Autodesk Inventor part; units mm, degrees
(part 2 of 2)
  line L957 (3.5682, -5.3852) -> (3.5463, -5.3913)
  line L958 (3.5463, -5.3913) -> (3.5215, -5.4036)
  line L959 (3.5215, -5.4036) -> (3.2974, -5.5433)
  line L960 (3.2974, -5.5433) -> (3.2248, -5.5858)
  line L961 (3.2248, -5.5858) -> (3.1517, -5.6274)
  line L962 (3.1517, -5.6274) -> (2.9187, -5.7518)
  line L963 (2.9187, -5.7518) -> (2.8957, -5.7671)
  line L964 (2.8957, -5.7671) -> (2.8794, -5.783)
  line L965 (2.8794, -5.783) -> (2.8651, -5.8021)
  line L966 (2.8651, -5.8021) -> (2.8529, -5.8243)
  line L967 (2.8529, -5.8243) -> (2.843, -5.8495)
  line L968 (2.843, -5.8495) -> (2.8303, -5.9087)
  line L969 (2.8303, -5.9087) -> (2.8281, -5.9788)
  line L970 (2.8281, -5.9788) -> (2.8371, -6.0592)
  line L971 (2.8371, -6.0592) -> (2.8582, -6.1489)
  line L972 (2.8582, -6.1489) -> (2.8922, -6.2471)
  line L973 (2.8922, -6.2471) -> (2.9398, -6.3529)
  line L974 (2.9398, -6.3529) -> (2.9659, -6.4039)
  line L975 (2.9659, -6.4039) -> (2.9967, -6.501)
  line L976 (2.9967, -6.501) -> (3.0239, -6.628)
  line L977 (3.0239, -6.628) -> (3.0364, -6.7098)
  line L978 (3.0364, -6.7098) -> (3.0468, -6.8051)
  line L979 (3.0468, -6.8051) -> (3.0541, -6.9129)
  line L980 (3.0541, -6.9129) -> (3.0571, -7.033)
  line L981 (3.0571, -7.033) -> (3.0548, -7.1683)
  line L982 (3.0548, -7.1683) -> (3.0464, -7.3121)
  line L983 (3.0464, -7.3121) -> (3.0306, -7.4689)
  line L984 (3.0306, -7.4689) -> (3.0065, -7.6369)
  line L985 (3.0065, -7.6369) -> (2.9731, -7.8164)
  line L986 (2.9731, -7.8164) -> (2.9366, -7.9766)
  arc A18 (2.3128, -8.1793) -> (2.9366, -7.9766) centre (0, 0) ccw
  line L987 (2.3128, -8.1793) -> (2.1908, -8.0711)
  line L988 (2.1908, -8.0711) -> (2.0582, -7.9456)
  line L989 (2.0582, -7.9456) -> (1.94, -7.8238)
  line L990 (1.94, -7.8238) -> (1.835, -7.7062)
  line L991 (1.835, -7.7062) -> (1.7437, -7.5949)
  line L992 (1.7437, -7.5949) -> (1.6623, -7.4867)
  line L993 (1.6623, -7.4867) -> (1.5942, -7.3878)
  line L994 (1.5942, -7.3878) -> (1.5367, -7.2963)
  line L995 (1.5367, -7.2963) -> (1.4891, -7.2131)
  line L996 (1.4891, -7.2131) -> (1.4511, -7.1396)
  line L997 (1.4511, -7.1396) -> (1.3985, -7.0209)
  line L998 (1.3985, -7.0209) -> (1.3663, -6.9242)
  line L999 (1.3663, -6.9242) -> (1.3573, -6.8676)
  line L1000 (1.3573, -6.8676) -> (1.3337, -6.754)
  line L1001 (1.3337, -6.754) -> (1.3034, -6.6546)
  line L1002 (1.3034, -6.6546) -> (1.2678, -6.5696)
  line L1003 (1.2678, -6.5696) -> (1.2278, -6.4993)
  line L1004 (1.2278, -6.4993) -> (1.1847, -6.4439)
  line L1005 (1.1847, -6.4439) -> (1.1397, -6.4035)
  line L1006 (1.1397, -6.4035) -> (1.1169, -6.389)
  line L1007 (1.1169, -6.389) -> (1.094, -6.3782)
  line L1008 (1.094, -6.3782) -> (1.0712, -6.3711)
  line L1009 (1.0712, -6.3711) -> (1.0486, -6.3678)
  line L1010 (1.0486, -6.3678) -> (1.021, -6.369)
  line L1011 (1.021, -6.369) -> (0.7594, -6.4054)
  line L1012 (0.7594, -6.4054) -> (0.6758, -6.4147)
  line L1013 (0.6758, -6.4147) -> (0.5922, -6.423)
  line L1014 (0.5922, -6.423) -> (0.3287, -6.4418)
  line L1015 (0.3287, -6.4418) -> (0.3014, -6.4464)
  line L1016 (0.3014, -6.4464) -> (0.2801, -6.4543)
  line L1017 (0.2801, -6.4543) -> (0.2592, -6.4659)
  line L1018 (0.2592, -6.4659) -> (0.2391, -6.4813)
  line L1019 (0.2391, -6.4813) -> (0.2197, -6.5002)
  line L1020 (0.2197, -6.5002) -> (0.1841, -6.5491)
  line L1021 (0.1841, -6.5491) -> (0.1535, -6.6123)
  line L1022 (0.1535, -6.6123) -> (0.1291, -6.6893)
  line L1023 (0.1291, -6.6893) -> (0.1119, -6.7799)
  line L1024 (0.1119, -6.7799) -> (0.103, -6.8834)
  line L1025 (0.103, -6.8834) -> (0.1034, -6.9994)
  line L1026 (0.1034, -6.9994) -> (0.1065, -7.0567)
  line L1027 (0.1065, -7.0567) -> (0.0951, -7.1579)
  line L1028 (0.0951, -7.1579) -> (0.0683, -7.285)
  line L1029 (0.0683, -7.285) -> (0.0464, -7.3648)
  line L1030 (0.0464, -7.3648) -> (0.0172, -7.4561)
  line L1031 (0.0172, -7.4561) -> (-0.02, -7.5575)
  line L1032 (-0.02, -7.5575) -> (-0.0661, -7.6685)
  line L1033 (-0.0661, -7.6685) -> (-0.1232, -7.7912)
  line L1034 (-0.1232, -7.7912) -> (-0.1894, -7.919)
  line L1035 (-0.1894, -7.919) -> (-0.2676, -8.0559)
  line L1036 (-0.2676, -8.0559) -> (-0.3579, -8.1996)
  line L1037 (-0.3579, -8.1996) -> (-0.4615, -8.35)
  line L1038 (-0.4615, -8.35) -> (-0.5599, -8.4815)
  arc A19 (-1.2139, -8.4129) -> (-0.5599, -8.4815) centre (0, 0) ccw
  line L1039 (-1.2139, -8.4129) -> (-1.283, -8.2636)
  line L1040 (-1.283, -8.2636) -> (-1.353, -8.0949)
  line L1041 (-1.353, -8.0949) -> (-1.4115, -7.9356)
  line L1042 (-1.4115, -7.9356) -> (-1.4595, -7.7855)
  line L1043 (-1.4595, -7.7855) -> (-1.4977, -7.6466)
  line L1044 (-1.4977, -7.6466) -> (-1.528, -7.5147)
  line L1045 (-1.528, -7.5147) -> (-1.55, -7.3966)
  line L1046 (-1.55, -7.3966) -> (-1.5653, -7.2897)
  line L1047 (-1.5653, -7.2897) -> (-1.5749, -7.1943)
  line L1048 (-1.5749, -7.1943) -> (-1.5798, -7.1116)
  line L1049 (-1.5798, -7.1116) -> (-1.5796, -6.9818)
  line L1050 (-1.5796, -6.9818) -> (-1.5697, -6.8804)
  line L1051 (-1.5697, -6.8804) -> (-1.5548, -6.8251)
  line L1052 (-1.5548, -6.8251) -> (-1.5302, -6.7117)
  line L1053 (-1.5302, -6.7117) -> (-1.5174, -6.6086)
  line L1054 (-1.5174, -6.6086) -> (-1.5154, -6.5164)
  line L1055 (-1.5154, -6.5164) -> (-1.5234, -6.4359)
  line L1056 (-1.5234, -6.4359) -> (-1.5402, -6.3678)
  line L1057 (-1.5402, -6.3678) -> (-1.5649, -6.3126)
  line L1058 (-1.5649, -6.3126) -> (-1.5798, -6.29)
  line L1059 (-1.5798, -6.29) -> (-1.5964, -6.2708)
  line L1060 (-1.5964, -6.2708) -> (-1.6143, -6.2551)
  line L1061 (-1.6143, -6.2551) -> (-1.6336, -6.2429)
  line L1062 (-1.6336, -6.2429) -> (-1.6593, -6.2328)
  line L1063 (-1.6593, -6.2328) -> (-1.9131, -6.1596)
  line L1064 (-1.9131, -6.1596) -> (-1.9932, -6.1342)
  line L1065 (-1.9932, -6.1342) -> (-2.073, -6.1077)
  line L1066 (-2.073, -6.1077) -> (-2.3214, -6.0177)
  line L1067 (-2.3214, -6.0177) -> (-2.3482, -6.0109)
  line L1068 (-2.3482, -6.0109) -> (-2.3709, -6.0094)
  line L1069 (-2.3709, -6.0094) -> (-2.3947, -6.0116)
  line L1070 (-2.3947, -6.0116) -> (-2.4193, -6.0174)
  line L1071 (-2.4193, -6.0174) -> (-2.4447, -6.0269)
  line L1072 (-2.4447, -6.0269) -> (-2.4971, -6.057)
  line L1073 (-2.4971, -6.057) -> (-2.5507, -6.1023)
  line L1074 (-2.5507, -6.1023) -> (-2.6044, -6.1627)
  line L1075 (-2.6044, -6.1627) -> (-2.657, -6.2385)
  line L1076 (-2.657, -6.2385) -> (-2.7072, -6.3295)
  line L1077 (-2.7072, -6.3295) -> (-2.7539, -6.4356)
  line L1078 (-2.7539, -6.4356) -> (-2.7745, -6.4891)
  line L1079 (-2.7745, -6.4891) -> (-2.826, -6.577)
  line L1080 (-2.826, -6.577) -> (-2.9021, -6.6822)
  line L1081 (-2.9021, -6.6822) -> (-2.9546, -6.7462)
  line L1082 (-2.9546, -6.7462) -> (-3.0185, -6.8178)
  line L1083 (-3.0185, -6.8178) -> (-3.0937, -6.8953)
  line L1084 (-3.0937, -6.8953) -> (-3.1809, -6.9779)
  line L1085 (-3.1809, -6.9779) -> (-3.283, -7.0668)
  line L1086 (-3.283, -7.0668) -> (-3.3955, -7.1566)
  line L1087 (-3.3955, -7.1566) -> (-3.5226, -7.2499)
  line L1088 (-3.5226, -7.2499) -> (-3.6636, -7.3444)
  line L1089 (-3.6636, -7.3444) -> (-3.8194, -7.4396)
  line L1090 (-3.8194, -7.4396) -> (-3.9628, -7.5197)
  arc A20 (-4.5309, -7.1917) -> (-3.9628, -7.5197) centre (0, 0) ccw
  line L1091 (-4.5309, -7.1917) -> (-4.5332, -7.0275)
  line L1092 (-4.5332, -7.0275) -> (-4.5286, -6.8449)
  line L1093 (-4.5286, -6.8449) -> (-4.5172, -6.6756)
  line L1094 (-4.5172, -6.6756) -> (-4.5001, -6.5189)
  line L1095 (-4.5001, -6.5189) -> (-4.4785, -6.3766)
  line L1096 (-4.4785, -6.3766) -> (-4.4526, -6.2437)
  line L1097 (-4.4526, -6.2437) -> (-4.4246, -6.1269)
  line L1098 (-4.4246, -6.1269) -> (-4.3951, -6.023)
  line L1099 (-4.3951, -6.023) -> (-4.3651, -5.9319)
  line L1100 (-4.3651, -5.9319) -> (-4.3359, -5.8544)
  line L1101 (-4.3359, -5.8544) -> (-4.2829, -5.7359)
  line L1102 (-4.2829, -5.7359) -> (-4.2326, -5.6473)
  line L1103 (-4.2326, -5.6473) -> (-4.1965, -5.6028)
  line L1104 (-4.1965, -5.6028) -> (-4.1279, -5.5092)
  line L1105 (-4.1279, -5.5092) -> (-4.0742, -5.4202)
  line L1106 (-4.0742, -5.4202) -> (-4.035, -5.3369)
  line L1107 (-4.035, -5.3369) -> (-4.0094, -5.2601)
  line L1108 (-4.0094, -5.2601) -> (-3.9971, -5.1911)
  line L1109 (-3.9971, -5.1911) -> (-3.9966, -5.1312)
  line L1110 (-3.9966, -5.1312) -> (-4.001, -5.1045)
  line L1111 (-4.001, -5.1045) -> (-4.0083, -5.0803)
  line L1112 (-4.0083, -5.0803) -> (-4.0184, -5.0586)
  line L1113 (-4.0184, -5.0586) -> (-4.031, -5.0396)
  line L1114 (-4.031, -5.0396) -> (-4.0503, -5.0199)
  line L1115 (-4.0503, -5.0199) -> (-4.2524, -4.8498)
  line L1116 (-4.2524, -4.8498) -> (-4.3153, -4.794)
  line L1117 (-4.3153, -4.794) -> (-4.3774, -4.7373)
  line L1118 (-4.3774, -4.7373) -> (-4.5677, -4.5541)
  line L1119 (-4.5677, -4.5541) -> (-4.5893, -4.5369)
  line L1120 (-4.5893, -4.5369) -> (-4.6095, -4.5264)
  line L1121 (-4.6095, -4.5264) -> (-4.6321, -4.5187)
  line L1122 (-4.6321, -4.5187) -> (-4.657, -4.5139)
  line L1123 (-4.657, -4.5139) -> (-4.684, -4.5123)
  line L1124 (-4.684, -4.5123) -> (-4.7442, -4.5185)
  line L1125 (-4.7442, -4.5185) -> (-4.8116, -4.538)
  line L1126 (-4.8116, -4.538) -> (-4.8852, -4.5714)
  line L1127 (-4.8852, -4.5714) -> (-4.964, -4.6192)
  line L1128 (-4.964, -4.6192) -> (-5.0469, -4.6819)
  line L1129 (-5.0469, -4.6819) -> (-5.1328, -4.7599)
  line L1130 (-5.1328, -4.7599) -> (-5.1733, -4.8004)
  line L1131 (-5.1733, -4.8004) -> (-5.2562, -4.8597)
  line L1132 (-5.2562, -4.8597) -> (-5.3685, -4.9249)
  line L1133 (-5.3685, -4.9249) -> (-5.4425, -4.962)
  line L1134 (-5.4425, -4.962) -> (-5.5299, -5.0014)
  line L1135 (-5.5299, -5.0014) -> (-5.6301, -5.0416)
  line L1136 (-5.6301, -5.0416) -> (-5.7434, -5.0816)
  line L1137 (-5.7434, -5.0816) -> (-5.8728, -5.1213)
  line L1138 (-5.8728, -5.1213) -> (-6.0121, -5.1577)
  line L1139 (-6.0121, -5.1577) -> (-6.1662, -5.1911)
  line L1140 (-6.1662, -5.1911) -> (-6.3334, -5.2201)
  line L1141 (-6.3334, -5.2201) -> (-6.5144, -5.2438)
  line L1142 (-6.5144, -5.2438) -> (-6.678, -5.2587)
  arc A21 (-7.0642, -4.7273) -> (-6.678, -5.2587) centre (0, 0) ccw
  line L1143 (-7.0642, -4.7273) -> (-6.9995, -4.5763)
  line L1144 (-6.9995, -4.5763) -> (-6.9211, -4.4114)
  line L1145 (-6.9211, -4.4114) -> (-6.8418, -4.2613)
  line L1146 (-6.8418, -4.2613) -> (-6.7625, -4.1251)
  line L1147 (-6.7625, -4.1251) -> (-6.6849, -4.0039)
  line L1148 (-6.6849, -4.0039) -> (-6.6071, -3.893)
  line L1149 (-6.6071, -3.893) -> (-6.5341, -3.7977)
  line L1150 (-6.5341, -3.7977) -> (-6.4649, -3.7147)
  line L1151 (-6.4649, -3.7147) -> (-6.4005, -3.6437)
  line L1152 (-6.4005, -3.6437) -> (-6.3423, -3.5848)
  line L1153 (-6.3423, -3.5848) -> (-6.2457, -3.4981)
  line L1154 (-6.2457, -3.4981) -> (-6.1637, -3.4376)
  line L1155 (-6.1637, -3.4376) -> (-6.1126, -3.4116)
  line L1156 (-6.1126, -3.4116) -> (-6.0119, -3.354)
  line L1157 (-6.0119, -3.354) -> (-5.9267, -3.2945)
  line L1158 (-5.9267, -3.2945) -> (-5.8569, -3.2343)
  line L1159 (-5.8569, -3.2343) -> (-5.8024, -3.1746)
  line L1160 (-5.8024, -3.1746) -> (-5.763, -3.1165)
  line L1161 (-5.763, -3.1165) -> (-5.7385, -3.0612)
  line L1162 (-5.7385, -3.0612) -> (-5.7317, -3.035)
  line L1163 (-5.7317, -3.035) -> (-5.7285, -3.0099)
  line L1164 (-5.7285, -3.0099) -> (-5.7287, -2.9859)
  line L1165 (-5.7287, -2.9859) -> (-5.7325, -2.9634)
  line L1166 (-5.7325, -2.9634) -> (-5.7421, -2.9375)
  line L1167 (-5.7421, -2.9375) -> (-5.8576, -2.7)
  line L1168 (-5.8576, -2.7) -> (-5.8923, -2.6234)
  line L1169 (-5.8923, -2.6234) -> (-5.9261, -2.5464)
  line L1170 (-5.9261, -2.5464) -> (-6.0254, -2.3016)
  line L1171 (-6.0254, -2.3016) -> (-6.0382, -2.2771)
  line L1172 (-6.0382, -2.2771) -> (-6.0523, -2.2593)
  line L1173 (-6.0523, -2.2593) -> (-6.0698, -2.243)
  line L1174 (-6.0698, -2.243) -> (-6.0906, -2.2286)
  line L1175 (-6.0906, -2.2286) -> (-6.1147, -2.2161)
  line L1176 (-6.1147, -2.2161) -> (-6.1721, -2.1973)
  line L1177 (-6.1721, -2.1973) -> (-6.2417, -2.1877)
  line L1178 (-6.2417, -2.1877) -> (-6.3225, -2.1883)
  line L1179 (-6.3225, -2.1883) -> (-6.414, -2.1999)
  line L1180 (-6.414, -2.1999) -> (-6.5152, -2.2235)
  line L1181 (-6.5152, -2.2235) -> (-6.6254, -2.2598)
  line L1182 (-6.6254, -2.2598) -> (-6.6789, -2.2803)
  line L1183 (-6.6789, -2.2803) -> (-6.7787, -2.3008)
  line L1184 (-6.7787, -2.3008) -> (-6.9078, -2.3146)
  line L1185 (-6.9078, -2.3146) -> (-6.9905, -2.3184)
  line L1186 (-6.9905, -2.3184) -> (-7.0864, -2.3188)
  line L1187 (-7.0864, -2.3188) -> (-7.1943, -2.3148)
  line L1188 (-7.1943, -2.3148) -> (-7.314, -2.3053)
  line L1189 (-7.314, -2.3053) -> (-7.4484, -2.2889)
  line L1190 (-7.4484, -2.2889) -> (-7.5904, -2.2654)
  line L1191 (-7.5904, -2.2654) -> (-7.7448, -2.2333)
  line L1192 (-7.7448, -2.2333) -> (-7.9093, -2.1918)
  line L1193 (-7.9093, -2.1918) -> (-8.0844, -2.1398)
  line L1194 (-8.0844, -2.1398) -> (-8.2399, -2.0868)
  arc A22 (-8.3763, -1.4451) -> (-8.2399, -2.0868) centre (0, 0) ccw
  line L1195 (-8.3763, -1.4451) -> (-8.2557, -1.3335)
  line L1196 (-8.2557, -1.3335) -> (-8.117, -1.2148)
  line L1197 (-8.117, -1.2148) -> (-7.9836, -1.1099)
  line L1198 (-7.9836, -1.1099) -> (-7.8556, -1.0178)
  line L1199 (-7.8556, -1.0178) -> (-7.7354, -0.9386)
  line L1200 (-7.7354, -0.9386) -> (-7.6193, -0.8689)
  line L1201 (-7.6193, -0.8689) -> (-7.5138, -0.8115)
  line L1202 (-7.5138, -0.8115) -> (-7.4169, -0.7639)
  line L1203 (-7.4169, -0.7639) -> (-7.3291, -0.7253)
  line L1204 (-7.3291, -0.7253) -> (-7.252, -0.6951)
  line L1205 (-7.252, -0.6951) -> (-7.1285, -0.6552)
  line L1206 (-7.1285, -0.6552) -> (-7.0289, -0.6334)
  line L1207 (-7.0289, -0.6334) -> (-6.9717, -0.6304)
  line L1208 (-6.9717, -0.6304) -> (-6.8563, -0.6188)
  line L1209 (-6.8563, -0.6188) -> (-6.7542, -0.5991)
  line L1210 (-6.7542, -0.5991) -> (-6.666, -0.5725)
  line L1211 (-6.666, -0.5725) -> (-6.5919, -0.5401)
  line L1212 (-6.5919, -0.5401) -> (-6.5323, -0.5031)
  line L1213 (-6.5323, -0.5031) -> (-6.4874, -0.4625)
  line L1214 (-6.4874, -0.4625) -> (-6.4705, -0.4413)
  line L1215 (-6.4705, -0.4413) -> (-6.4574, -0.4197)
  line L1216 (-6.4574, -0.4197) -> (-6.448, -0.3977)
  line L1217 (-6.448, -0.3977) -> (-6.4424, -0.3757)
  line L1218 (-6.4424, -0.3757) -> (-6.4406, -0.3481)
  line L1219 (-6.4406, -0.3481) -> (-6.4495, -0.0841)
  line L1220 (-6.4495, -0.0841) -> (-6.45, 0)
  line L1221 (-6.45, 0) -> (-6.4495, 0.0841)
  line L1222 (-6.4495, 0.0841) -> (-6.4406, 0.3481)
  line L1223 (-6.4406, 0.3481) -> (-6.4423, 0.3756)
  line L1224 (-6.4423, 0.3756) -> (-6.448, 0.3977)
  line L1225 (-6.448, 0.3977) -> (-6.4574, 0.4196)
  line L1226 (-6.4574, 0.4196) -> (-6.4705, 0.4413)
  line L1227 (-6.4705, 0.4413) -> (-6.4873, 0.4625)
  line L1228 (-6.4873, 0.4625) -> (-6.5322, 0.503)
  line L1229 (-6.5322, 0.503) -> (-6.5918, 0.5401)
  line L1230 (-6.5918, 0.5401) -> (-6.6659, 0.5725)
  line L1231 (-6.6659, 0.5725) -> (-6.7542, 0.5991)
  line L1232 (-6.7542, 0.5991) -> (-6.8562, 0.6187)
  line L1233 (-6.8562, 0.6187) -> (-6.9716, 0.6303)
  line L1234 (-6.9716, 0.6303) -> (-7.0289, 0.6333)
  line L1235 (-7.0289, 0.6333) -> (-7.1284, 0.6552)
  line L1236 (-7.1284, 0.6552) -> (-7.2519, 0.6951)
  line L1237 (-7.2519, 0.6951) -> (-7.3291, 0.7253)
  line L1238 (-7.3291, 0.7253) -> (-7.4168, 0.7639)
  line L1239 (-7.4168, 0.7639) -> (-7.5138, 0.8115)
  line L1240 (-7.5138, 0.8115) -> (-7.6193, 0.8689)
  line L1241 (-7.6193, 0.8689) -> (-7.7354, 0.9385)
  line L1242 (-7.7354, 0.9385) -> (-7.8556, 1.0177)
  line L1243 (-7.8556, 1.0177) -> (-7.9836, 1.1098)
  line L1244 (-7.9836, 1.1098) -> (-8.117, 1.2146)
  line L1245 (-8.117, 1.2146) -> (-8.2558, 1.3333)
  line L1246 (-8.2558, 1.3333) -> (-8.3763, 1.445)
  arc A23 (-8.2401, 2.0859) -> (-8.3763, 1.445) centre (0, 0) ccw
  line L1247 (-8.2401, 2.0859) -> (-8.0846, 2.1389)
  line L1248 (-8.0846, 2.1389) -> (-7.9096, 2.1909)
  line L1249 (-7.9096, 2.1909) -> (-7.745, 2.2324)
  line L1250 (-7.745, 2.2324) -> (-7.5907, 2.2646)
  line L1251 (-7.5907, 2.2646) -> (-7.4486, 2.288)
  line L1252 (-7.4486, 2.288) -> (-7.3143, 2.3045)
  line L1253 (-7.3143, 2.3045) -> (-7.1945, 2.314)
  line L1254 (-7.1945, 2.314) -> (-7.0866, 2.3181)
  line L1255 (-7.0866, 2.3181) -> (-6.9907, 2.3177)
  line L1256 (-6.9907, 2.3177) -> (-6.908, 2.3139)
  line L1257 (-6.908, 2.3139) -> (-6.7789, 2.3001)
  line L1258 (-6.7789, 2.3001) -> (-6.6791, 2.2796)
  line L1259 (-6.6791, 2.2796) -> (-6.6256, 2.2591)
  line L1260 (-6.6256, 2.2591) -> (-6.5154, 2.2228)
  line L1261 (-6.5154, 2.2228) -> (-6.4142, 2.1992)
  line L1262 (-6.4142, 2.1992) -> (-6.3228, 2.1876)
  line L1263 (-6.3228, 2.1876) -> (-6.2419, 2.1871)
  line L1264 (-6.2419, 2.1871) -> (-6.1724, 2.1967)
  line L1265 (-6.1724, 2.1967) -> (-6.1149, 2.2155)
  line L1266 (-6.1149, 2.2155) -> (-6.0909, 2.228)
  line L1267 (-6.0909, 2.228) -> (-6.0701, 2.2424)
  line L1268 (-6.0701, 2.2424) -> (-6.0526, 2.2587)
  line L1269 (-6.0526, 2.2587) -> (-6.0385, 2.2765)
  line L1270 (-6.0385, 2.2765) -> (-6.0256, 2.301)
  line L1271 (-6.0256, 2.301) -> (-5.9264, 2.5458)
  line L1272 (-5.9264, 2.5458) -> (-5.8927, 2.6228)
  line L1273 (-5.8927, 2.6228) -> (-5.858, 2.6994)
  line L1274 (-5.858, 2.6994) -> (-5.7425, 2.937)
  line L1275 (-5.7425, 2.937) -> (-5.7329, 2.9629)
  line L1276 (-5.7329, 2.9629) -> (-5.7291, 2.9854)
  line L1277 (-5.7291, 2.9854) -> (-5.7288, 3.0092)
  line L1278 (-5.7288, 3.0092) -> (-5.732, 3.0343)
  line L1279 (-5.732, 3.0343) -> (-5.7388, 3.0606)
  line L1280 (-5.7388, 3.0606) -> (-5.7633, 3.1158)
  line L1281 (-5.7633, 3.1158) -> (-5.8027, 3.1739)
  line L1282 (-5.8027, 3.1739) -> (-5.8572, 3.2336)
  line L1283 (-5.8572, 3.2336) -> (-5.927, 3.2938)
  line L1284 (-5.927, 3.2938) -> (-6.0122, 3.3533)
  line L1285 (-6.0122, 3.3533) -> (-6.113, 3.4108)
  line L1286 (-6.113, 3.4108) -> (-6.164, 3.4368)
  line L1287 (-6.164, 3.4368) -> (-6.2461, 3.4973)
  line L1288 (-6.2461, 3.4973) -> (-6.3427, 3.584)
  line L1289 (-6.3427, 3.584) -> (-6.4009, 3.6429)
  line L1290 (-6.4009, 3.6429) -> (-6.4653, 3.7139)
  line L1291 (-6.4653, 3.7139) -> (-6.5346, 3.7968)
  line L1292 (-6.5346, 3.7968) -> (-6.6076, 3.8921)
  line L1293 (-6.6076, 3.8921) -> (-6.6853, 4.003)
  line L1294 (-6.6853, 4.003) -> (-6.763, 4.1242)
  line L1295 (-6.763, 4.1242) -> (-6.8424, 4.2604)
  line L1296 (-6.8424, 4.2604) -> (-6.9217, 4.4104)
  line L1297 (-6.9217, 4.4104) -> (-7.0001, 4.5753)
  line L1298 (-7.0001, 4.5753) -> (-7.0648, 4.7263)
  arc A24 (-6.6793, 5.2571) -> (-7.0648, 4.7263) centre (0, 0) ccw
  line L1299 (-6.6793, 5.2571) -> (-6.5157, 5.2423)
  line L1300 (-6.5157, 5.2423) -> (-6.3346, 5.2186)
  line L1301 (-6.3346, 5.2186) -> (-6.1674, 5.1896)
  line L1302 (-6.1674, 5.1896) -> (-6.0133, 5.1562)
  line L1303 (-6.0133, 5.1562) -> (-5.874, 5.1199)
  line L1304 (-5.874, 5.1199) -> (-5.7446, 5.0802)
  line L1305 (-5.7446, 5.0802) -> (-5.6313, 5.0402)
  line L1306 (-5.6313, 5.0402) -> (-5.5311, 5)
  line L1307 (-5.5311, 5) -> (-5.4437, 4.9607)
  line L1308 (-5.4437, 4.9607) -> (-5.3696, 4.9236)
  line L1309 (-5.3696, 4.9236) -> (-5.2573, 4.8585)
  line L1310 (-5.2573, 4.8585) -> (-5.1745, 4.7992)
  line L1311 (-5.1745, 4.7992) -> (-5.1339, 4.7586)
  line L1312 (-5.1339, 4.7586) -> (-5.0481, 4.6807)
  line L1313 (-5.0481, 4.6807) -> (-4.9651, 4.618)
  line L1314 (-4.9651, 4.618) -> (-4.8863, 4.5702)
  line L1315 (-4.8863, 4.5702) -> (-4.8127, 4.5368)
  line L1316 (-4.8127, 4.5368) -> (-4.7453, 4.5173)
  line L1317 (-4.7453, 4.5173) -> (-4.6851, 4.5111)
  line L1318 (-4.6851, 4.5111) -> (-4.6581, 4.5127)
  line L1319 (-4.6581, 4.5127) -> (-4.6332, 4.5175)
  line L1320 (-4.6332, 4.5175) -> (-4.6106, 4.5252)
  line L1321 (-4.6106, 4.5252) -> (-4.5904, 4.5357)
  line L1322 (-4.5904, 4.5357) -> (-4.5688, 4.5529)
  line L1323 (-4.5688, 4.5529) -> (-4.3785, 4.7361)
  line L1324 (-4.3785, 4.7361) -> (-4.3164, 4.7928)
  line L1325 (-4.3164, 4.7928) -> (-4.2535, 4.8486)
  line L1326 (-4.2535, 4.8486) -> (-4.0514, 5.0187)
  line L1327 (-4.0514, 5.0187) -> (-4.0321, 5.0385)
  line L1328 (-4.0321, 5.0385) -> (-4.0195, 5.0574)
  line L1329 (-4.0195, 5.0574) -> (-4.0095, 5.0791)
  line L1330 (-4.0095, 5.0791) -> (-4.0021, 5.1033)
  line L1331 (-4.0021, 5.1033) -> (-3.9977, 5.13)
  line L1332 (-3.9977, 5.13) -> (-3.9977, 5.1906)
  line L1333 (-3.9977, 5.1906) -> (-4.01, 5.2597)
  line L1334 (-4.01, 5.2597) -> (-4.0355, 5.3364)
  line L1335 (-4.0355, 5.3364) -> (-4.0748, 5.4198)
  line L1336 (-4.0748, 5.4198) -> (-4.1285, 5.5088)
  line L1337 (-4.1285, 5.5088) -> (-4.1971, 5.6024)
  line L1338 (-4.1971, 5.6024) -> (-4.2331, 5.6469)
  line L1339 (-4.2331, 5.6469) -> (-4.2835, 5.7355)
  line L1340 (-4.2835, 5.7355) -> (-4.3365, 5.854)
  line L1341 (-4.3365, 5.854) -> (-4.3657, 5.9315)
  line L1342 (-4.3657, 5.9315) -> (-4.3957, 6.0226)
  line L1343 (-4.3957, 6.0226) -> (-4.4252, 6.1265)
  line L1344 (-4.4252, 6.1265) -> (-4.4532, 6.2433)
  line L1345 (-4.4532, 6.2433) -> (-4.4791, 6.3761)
  line L1346 (-4.4791, 6.3761) -> (-4.5007, 6.5185)
  line L1347 (-4.5007, 6.5185) -> (-4.5179, 6.6752)
  line L1348 (-4.5179, 6.6752) -> (-4.5292, 6.8445)
  line L1349 (-4.5292, 6.8445) -> (-4.5339, 7.0271)
  line L1350 (-4.5339, 7.0271) -> (-4.5316, 7.1913)
  arc A25 (-3.9636, 7.5193) -> (-4.5316, 7.1913) centre (0, 0) ccw
  line L1351 (-3.9636, 7.5193) -> (-3.8201, 7.4392)
  line L1352 (-3.8201, 7.4392) -> (-3.6644, 7.344)
  line L1353 (-3.6644, 7.344) -> (-3.5234, 7.2495)
  line L1354 (-3.5234, 7.2495) -> (-3.3963, 7.1563)
  line L1355 (-3.3963, 7.1563) -> (-3.2838, 7.0664)
  line L1356 (-3.2838, 7.0664) -> (-3.1817, 6.9775)
  line L1357 (-3.1817, 6.9775) -> (-3.0945, 6.8949)
  line L1358 (-3.0945, 6.8949) -> (-3.0193, 6.8174)
  line L1359 (-3.0193, 6.8174) -> (-2.9554, 6.7458)
  line L1360 (-2.9554, 6.7458) -> (-2.9029, 6.6818)
  line L1361 (-2.9029, 6.6818) -> (-2.8268, 6.5767)
  line L1362 (-2.8268, 6.5767) -> (-2.7753, 6.4887)
  line L1363 (-2.7753, 6.4887) -> (-2.7547, 6.4352)
  line L1364 (-2.7547, 6.4352) -> (-2.708, 6.3291)
  line L1365 (-2.708, 6.3291) -> (-2.6578, 6.2381)
  line L1366 (-2.6578, 6.2381) -> (-2.6052, 6.1624)
  line L1367 (-2.6052, 6.1624) -> (-2.5515, 6.1019)
  line L1368 (-2.5515, 6.1019) -> (-2.4978, 6.0567)
  line L1369 (-2.4978, 6.0567) -> (-2.4454, 6.0265)
  line L1370 (-2.4454, 6.0265) -> (-2.42, 6.0171)
  line L1371 (-2.42, 6.0171) -> (-2.3954, 6.0113)
  line L1372 (-2.3954, 6.0113) -> (-2.3716, 6.0091)
  line L1373 (-2.3716, 6.0091) -> (-2.3489, 6.0106)
  line L1374 (-2.3489, 6.0106) -> (-2.3221, 6.0174)
  line L1375 (-2.3221, 6.0174) -> (-2.0738, 6.1075)
  line L1376 (-2.0738, 6.1075) -> (-1.994, 6.134)
  line L1377 (-1.994, 6.134) -> (-1.9139, 6.1594)
  line L1378 (-1.9139, 6.1594) -> (-1.6601, 6.2326)
  line L1379 (-1.6601, 6.2326) -> (-1.6344, 6.2428)
  line L1380 (-1.6344, 6.2428) -> (-1.6151, 6.255)
  line L1381 (-1.6151, 6.255) -> (-1.5972, 6.2707)
  line L1382 (-1.5972, 6.2707) -> (-1.5806, 6.2899)
  line L1383 (-1.5806, 6.2899) -> (-1.5657, 6.3125)
  line L1384 (-1.5657, 6.3125) -> (-1.541, 6.3677)
  line L1385 (-1.541, 6.3677) -> (-1.5242, 6.4358)
  line L1386 (-1.5242, 6.4358) -> (-1.5163, 6.5163)
  line L1387 (-1.5163, 6.5163) -> (-1.5183, 6.6084)
  line L1388 (-1.5183, 6.6084) -> (-1.5311, 6.7116)
  line L1389 (-1.5311, 6.7116) -> (-1.5557, 6.8249)
  line L1390 (-1.5557, 6.8249) -> (-1.5706, 6.8803)
  line L1391 (-1.5706, 6.8803) -> (-1.5805, 6.9817)
  line L1392 (-1.5805, 6.9817) -> (-1.5808, 7.1115)
  line L1393 (-1.5808, 7.1115) -> (-1.5759, 7.1942)
  line L1394 (-1.5759, 7.1942) -> (-1.5663, 7.2896)
  line L1395 (-1.5663, 7.2896) -> (-1.551, 7.3965)
  line L1396 (-1.551, 7.3965) -> (-1.529, 7.5146)
  line L1397 (-1.529, 7.5146) -> (-1.4987, 7.6465)
  line L1398 (-1.4987, 7.6465) -> (-1.4605, 7.7853)
  line L1399 (-1.4605, 7.7853) -> (-1.4125, 7.9355)
  line L1400 (-1.4125, 7.9355) -> (-1.354, 8.0948)
  line L1401 (-1.354, 8.0948) -> (-1.284, 8.2634)
  line L1402 (-1.284, 8.2634) -> (-1.2149, 8.4127)
  arc A26 (-0.5625, 8.4814) -> (-1.2149, 8.4127) centre (0, 0) ccw
  line L1403 (-0.5625, 8.4814) -> (-0.4641, 8.3499)
  line L1404 (-0.4641, 8.3499) -> (-0.3605, 8.1995)
  line L1405 (-0.3605, 8.1995) -> (-0.2702, 8.0558)
  line L1406 (-0.2702, 8.0558) -> (-0.1919, 7.919)
  line L1407 (-0.1919, 7.919) -> (-0.1257, 7.7911)
  line L1408 (-0.1257, 7.7911) -> (-0.0686, 7.6684)
  line L1409 (-0.0686, 7.6684) -> (-0.0225, 7.5575)
  line L1410 (-0.0225, 7.5575) -> (0.0147, 7.4561)
  line L1411 (0.0147, 7.4561) -> (0.0439, 7.3648)
  line L1412 (0.0439, 7.3648) -> (0.0659, 7.2849)
  line L1413 (0.0659, 7.2849) -> (0.0926, 7.1579)
  line L1414 (0.0926, 7.1579) -> (0.104, 7.0566)
  line L1415 (0.104, 7.0566) -> (0.101, 6.9994)
  line L1416 (0.101, 6.9994) -> (0.1005, 6.8834)
  line L1417 (0.1005, 6.8834) -> (0.1094, 6.7798)
  line L1418 (0.1094, 6.7798) -> (0.1266, 6.6893)
  line L1419 (0.1266, 6.6893) -> (0.1511, 6.6122)
  line L1420 (0.1511, 6.6122) -> (0.1817, 6.5491)
  line L1421 (0.1817, 6.5491) -> (0.2173, 6.5002)
  line L1422 (0.2173, 6.5002) -> (0.2366, 6.4812)
  line L1423 (0.2366, 6.4812) -> (0.2568, 6.4659)
  line L1424 (0.2568, 6.4659) -> (0.2776, 6.4543)
  line L1425 (0.2776, 6.4543) -> (0.299, 6.4463)
  line L1426 (0.299, 6.4463) -> (0.3262, 6.4417)
  line L1427 (0.3262, 6.4417) -> (0.5897, 6.4229)
  line L1428 (0.5897, 6.4229) -> (0.6734, 6.4146)
  line L1429 (0.6734, 6.4146) -> (0.7569, 6.4053)
  line L1430 (0.7569, 6.4053) -> (1.0186, 6.3689)
  line L1431 (1.0186, 6.3689) -> (1.0462, 6.3678)
  line L1432 (1.0462, 6.3678) -> (1.0687, 6.3711)
  line L1433 (1.0687, 6.3711) -> (1.0915, 6.3781)
  line L1434 (1.0915, 6.3781) -> (1.1144, 6.3889)
  line L1435 (1.1144, 6.3889) -> (1.1373, 6.4034)
  line L1436 (1.1373, 6.4034) -> (1.1823, 6.4438)
  line L1437 (1.1823, 6.4438) -> (1.2253, 6.4992)
  line L1438 (1.2253, 6.4992) -> (1.2653, 6.5695)
  line L1439 (1.2653, 6.5695) -> (1.301, 6.6545)
  line L1440 (1.301, 6.6545) -> (1.3312, 6.754)
  line L1441 (1.3312, 6.754) -> (1.3548, 6.8675)
  line L1442 (1.3548, 6.8675) -> (1.3638, 6.9241)
  line L1443 (1.3638, 6.9241) -> (1.396, 7.0208)
  line L1444 (1.396, 7.0208) -> (1.4486, 7.1395)
  line L1445 (1.4486, 7.1395) -> (1.4866, 7.2131)
  line L1446 (1.4866, 7.2131) -> (1.5342, 7.2963)
  line L1447 (1.5342, 7.2963) -> (1.5917, 7.3878)
  line L1448 (1.5917, 7.3878) -> (1.6598, 7.4867)
  line L1449 (1.6598, 7.4867) -> (1.7411, 7.5949)
  line L1450 (1.7411, 7.5949) -> (1.8324, 7.7062)
  line L1451 (1.8324, 7.7062) -> (1.9374, 7.8238)
  line L1452 (1.9374, 7.8238) -> (2.0556, 7.9456)
  line L1453 (2.0556, 7.9456) -> (2.1882, 8.0711)
  line L1454 (2.1882, 8.0711) -> (2.3119, 8.1796)
  arc A27 (2.9362, 7.9768) -> (2.3119, 8.1796) centre (0, 0) ccw
  line L1455 (2.9362, 7.9768) -> (2.9727, 7.8166)
  line L1456 (2.9727, 7.8166) -> (3.0061, 7.6371)
  line L1457 (3.0061, 7.6371) -> (3.0302, 7.4691)
  line L1458 (3.0302, 7.4691) -> (3.046, 7.3122)
  line L1459 (3.046, 7.3122) -> (3.0545, 7.1685)
  line L1460 (3.0545, 7.1685) -> (3.0568, 7.0332)
  line L1461 (3.0568, 7.0332) -> (3.0537, 6.9131)
  line L1462 (3.0537, 6.9131) -> (3.0465, 6.8053)
  line L1463 (3.0465, 6.8053) -> (3.0361, 6.71)
  line L1464 (3.0361, 6.71) -> (3.0237, 6.6281)
  line L1465 (3.0237, 6.6281) -> (2.9964, 6.5012)
  line L1466 (2.9964, 6.5012) -> (2.9656, 6.4041)
  line L1467 (2.9656, 6.4041) -> (2.9396, 6.353)
  line L1468 (2.9396, 6.353) -> (2.892, 6.2472)
  line L1469 (2.892, 6.2472) -> (2.858, 6.149)
  line L1470 (2.858, 6.149) -> (2.8369, 6.0593)
  line L1471 (2.8369, 6.0593) -> (2.8279, 5.9789)
  line L1472 (2.8279, 5.9789) -> (2.8302, 5.9088)
  line L1473 (2.8302, 5.9088) -> (2.8429, 5.8497)
  line L1474 (2.8429, 5.8497) -> (2.8528, 5.8244)
  line L1475 (2.8528, 5.8244) -> (2.865, 5.8022)
  line L1476 (2.865, 5.8022) -> (2.8793, 5.7832)
  line L1477 (2.8793, 5.7832) -> (2.8956, 5.7672)
  line L1478 (2.8956, 5.7672) -> (2.9186, 5.7519)
  line L1479 (2.9186, 5.7519) -> (3.1517, 5.6276)
  line L1480 (3.1517, 5.6276) -> (3.2248, 5.586)
  line L1481 (3.2248, 5.586) -> (3.2973, 5.5435)
  line L1482 (3.2973, 5.5435) -> (3.5215, 5.4039)
  line L1483 (3.5215, 5.4039) -> (3.5463, 5.3916)
  line L1484 (3.5463, 5.3916) -> (3.5682, 5.3855)
  line L1485 (3.5682, 5.3855) -> (3.5919, 5.3826)
  line L1486 (3.5919, 5.3826) -> (3.6172, 5.3832)
  line L1487 (3.6172, 5.3832) -> (3.644, 5.3872)
  line L1488 (3.644, 5.3872) -> (3.7016, 5.4058)
  line L1489 (3.7016, 5.4058) -> (3.7634, 5.4389)
  line L1490 (3.7634, 5.4389) -> (3.8285, 5.4869)
  line L1491 (3.8285, 5.4869) -> (3.8957, 5.55)
  line L1492 (3.8957, 5.55) -> (3.9637, 5.6286)
  line L1493 (3.9637, 5.6286) -> (4.0315, 5.7227)
  line L1494 (4.0315, 5.7227) -> (4.0627, 5.7708)
  line L1495 (4.0627, 5.7708) -> (4.1314, 5.846)
  line L1496 (4.1314, 5.846) -> (4.2277, 5.9331)
  line L1497 (4.2277, 5.9331) -> (4.2924, 5.9848)
  line L1498 (4.2924, 5.9848) -> (4.3697, 6.0414)
  line L1499 (4.3697, 6.0414) -> (4.4594, 6.1016)
  line L1500 (4.4594, 6.1016) -> (4.5619, 6.1643)
  line L1501 (4.5619, 6.1643) -> (4.6803, 6.23)
  line L1502 (4.6803, 6.23) -> (4.8089, 6.2946)
  line L1503 (4.8089, 6.2946) -> (4.9527, 6.3593)
  line L1504 (4.9527, 6.3593) -> (5.1102, 6.4225)
  line L1505 (5.1102, 6.4225) -> (5.2824, 6.4833)
  line L1506 (5.2824, 6.4833) -> (5.4393, 6.5318)
  arc A28 (5.9265, 6.0931) -> (5.4393, 6.5318) centre (0, 0) ccw
  line L1507 (5.9265, 6.0931) -> (5.8947, 5.932)
  line L1508 (5.8947, 5.932) -> (5.8523, 5.7544)
  line L1509 (5.8523, 5.7544) -> (5.8059, 5.5911)
  line L1510 (5.8059, 5.5911) -> (5.7566, 5.4414)
  line L1511 (5.7566, 5.4414) -> (5.7059, 5.3066)
  line L1512 (5.7059, 5.3066) -> (5.6529, 5.1821)
  line L1513 (5.6529, 5.1821) -> (5.6012, 5.0736)
  line L1514 (5.6012, 5.0736) -> (5.5508, 4.9781)
  line L1515 (5.5508, 4.9781) -> (5.5025, 4.8953)
  line L1516 (5.5025, 4.8953) -> (5.4579, 4.8255)
  line L1517 (5.4579, 4.8255) -> (5.3814, 4.7206)
  line L1518 (5.3814, 4.7206) -> (5.3137, 4.6444)
  line L1519 (5.3137, 4.6444) -> (5.2692, 4.6084)
  line L1520 (5.2692, 4.6084) -> (5.1827, 4.5311)
  line L1521 (5.1827, 4.5311) -> (5.1117, 4.4552)
  line L1522 (5.1117, 4.4552) -> (5.0559, 4.3818)
  line L1523 (5.0559, 4.3818) -> (5.015, 4.3121)
  line L1524 (5.015, 4.3121) -> (4.9885, 4.2471)
  line L1525 (4.9885, 4.2471) -> (4.976, 4.1879)
  line L1526 (4.976, 4.1879) -> (4.9749, 4.1608)
  line L1527 (4.9749, 4.1608) -> (4.977, 4.1356)
  line L1528 (4.977, 4.1356) -> (4.9823, 4.1123)
  line L1529 (4.9823, 4.1123) -> (4.9907, 4.0912)
  line L1530 (4.9907, 4.0912) -> (5.0054, 4.0678)
  line L1531 (5.0054, 4.0678) -> (5.1677, 3.8594)
  line L1532 (5.1677, 3.8594) -> (5.2176, 3.7917)
  line L1533 (5.2176, 3.7917) -> (5.2666, 3.7234)
  line L1534 (5.2666, 3.7234) -> (5.4145, 3.5045)
  line L1535 (5.4145, 3.5045) -> (5.4321, 3.4833)
  line L1536 (5.4321, 3.4833) -> (5.4497, 3.4687)
  line L1537 (5.4497, 3.4687) -> (5.4702, 3.4565)
  line L1538 (5.4702, 3.4565) -> (5.4935, 3.4467)
  line L1539 (5.4935, 3.4467) -> (5.5196, 3.4394)
  line L1540 (5.5196, 3.4394) -> (5.5797, 3.433)
  line L1541 (5.5797, 3.433) -> (5.6497, 3.4381)
  line L1542 (5.6497, 3.4381) -> (5.7287, 3.4554)
  line L1543 (5.7287, 3.4554) -> (5.8158, 3.4858)
  line L1544 (5.8158, 3.4858) -> (5.9099, 3.5298)
  line L1545 (5.9099, 3.5298) -> (6.0101, 3.5883)
  line L1546 (6.0101, 3.5883) -> (6.0581, 3.6195)
  line L1547 (6.0581, 3.6195) -> (6.1515, 3.6603)
  line L1548 (6.1515, 3.6603) -> (6.2749, 3.7006)
  line L1549 (6.2749, 3.7006) -> (6.355, 3.7216)
  line L1550 (6.355, 3.7216) -> (6.4487, 3.7419)
  line L1551 (6.4487, 3.7419) -> (6.5551, 3.7604)
  line L1552 (6.5551, 3.7604) -> (6.6742, 3.776)
  line L1553 (6.6742, 3.776) -> (6.8091, 3.7879)
  line L1554 (6.8091, 3.7879) -> (6.9529, 3.7945)
  line L1555 (6.9529, 3.7945) -> (7.1105, 3.7952)
  line L1556 (7.1105, 3.7952) -> (7.2801, 3.7888)
  line L1557 (7.2801, 3.7888) -> (7.4621, 3.7743)
  line L1558 (7.4621, 3.7743) -> (7.6256, 3.755)
  arc A29 (7.8928, 3.155) -> (7.6256, 3.755) centre (0, 0) ccw
  line L1559 (7.8928, 3.155) -> (7.7981, 3.0207)
  line L1560 (0, 3.4641) -> (3, 1.7321)
  line L1561 (3, 1.7321) -> (3, -1.7321)
  line L1562 (3, -1.7321) -> (0, -3.4641)
  line L1563 (0, -3.4641) -> (-3, -1.7321)
  line L1564 (-3, -1.7321) -> (-3, 1.7321)
  line L1565 (-3, 1.7321) -> (0, 3.4641)
  dimension "d0" = 6
  constraints: 3132 end point, 60 parallel, 60 perpendicular, 60 point on circle, 30 centre point, 21 concentric, 2 coincident, 1 vertical, 13 other
  measures "d0" distance of L1561.end L1563.end
extrude "Extrusión1" add sketch "Boceto1" along normal blind 6
